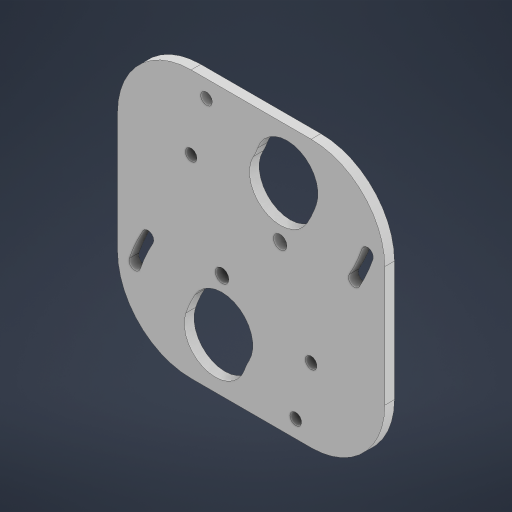
# Autodesk Inventor part: mount-plate
Saved by Autodesk Inventor 2024 (Build 280153000, 153)
## iProperties
Created: 2024-10-25
Part Number: mount-plate
Material: Generic
Document SubType Name: Modeling
Designer: loren
Density: 1 g/cm^3
Appearance: Default
Author: loren
## iProperties of the stored document mount-plate_3DPrint.ipt
Created: 2026-02-06
Part Number: mount-plate_3DPrint
Material: Generic
Document SubType Name: Modeling
Designer: lokies
Density: 1 g/cm^3
Appearance: Default
Author: lokies
Autodesk Inventor part; units mm, degrees
ref_plane "YZ Plane" through (0, 0, 0) normal (1, 0, 0) x (0, 1, 0)
ref_plane "XZ Plane" through (0, 0, 0) normal (0, 1, 0) x (-1, 0, 0)
ref_plane "XY Plane" through (0, 0, 0) normal (0, 0, 1) x (1, 0, 0)
sketch "Sketch1" plane through (0, 0, 0) normal (0, 1, 0) x (-1, 0, 0)
  line L0 (34.5, 34.5) -> (-34.5, 34.5)
  line L1 (-34.5, 34.5) -> (-34.5, -34.5)
  line L2 (-34.5, -34.5) -> (34.5, -34.5)
  line L3 (34.5, -34.5) -> (34.5, 34.5)
  point P0 (0, 0)
  point P1 (-34.5, 0)
  point P2 (0, 34.5)
  dimension "d0" = 69
  constraints: 8 end point, 2 midpoint, 2 parallel, 2 perpendicular, 1 horizontal, 1 horizontal alignment, 1 vertical alignment
  measures "d0" distance of L2.end L1.end
extrude "Extrusion1" add sketch "Sketch1" against normal blind 2.5
sketch "Sketch2" plane through (0, -2.5, 0) normal (0, -1, 0) x (1, 0, 0)
  circle A0 centre (-15.5, 15.5) radius 19.9 construction
  line L0 (-15.5, 15.5) -> (15.5, -15.5) construction
  circle A1 centre (-15.5, 15.5) radius 1.5
  circle A2 centre (-11.5216, 30.0556) radius 1.5
  line L1 (-11.5216, 30.0556) -> (28.9823, 13.2551) construction
  arc A3 (26.633, 8.4441) -> (30.0556, 16.1214) centre (-11.5216, 30.0556) ccw construction
  arc A4 (27.9381, 7.7048) -> (31.4779, 15.6448) centre (-11.5216, 30.0556) ccw
  arc A5 (25.3278, 9.1834) -> (28.6334, 16.5981) centre (-11.5216, 30.0556) ccw
  arc A6 (31.4779, 15.6448) -> (28.6334, 16.5981) centre (30.0556, 16.1214) ccw
  arc A7 (25.3278, 9.1834) -> (27.9381, 7.7048) centre (26.633, 8.4441) ccw
  arc A8 (7.5557, 19.2499) -> (9.267, 23.0885) centre (-11.5216, 30.0556) ccw construction
  arc A9 (16.8524, 20.5464) -> (1.6817, 25.6307) centre (9.267, 23.0885) ccw
  arc A10 (0.5948, 23.1927) -> (14.5166, 15.3071) centre (7.5557, 19.2499) ccw
  arc A11 (14.5166, 15.3071) -> (16.8524, 20.5464) centre (-11.5216, 30.0556) ccw
  arc A12 (0.5948, 23.1927) -> (1.6817, 25.6307) centre (-11.5216, 30.0556) ccw
  circle A13 centre (7.5557, 19.2499) radius 18.25 construction
  line L2 (-11.5216, 31.5556) -> (-11.5216, 34.5) construction
  line L3 (34.5, 34.5) -> (-34.5, 34.5) projected
  line L4 (31.5556, 16.1214) -> (34.5, 16.1214) construction
  line L5 (34.5, -34.5) -> (34.5, 34.5) projected
  line L6 (0, 0) -> (7.5, 7.5) construction
  circle A14 centre (7.5, 7.5) radius 1.75
  line L7 (7.5178, 11.25) -> (7.5083, 9.25) construction
  line L8 (-34.5, 34.5) -> (-34.5, -34.5) projected
  arc A15 (-15.5, 34.5) -> (-34.5, 15.5) centre (-15.5, 15.5) ccw
  arc A16 (34.5, 15.5) -> (15.5, 34.5) centre (15.5, 15.5) ccw
  point P0 (8.7304, 21.6553)
  dimension "d5" = 3
  dimension "d18" = 3.5
  dimension "d3" = 39.8
  dimension "d4" = 3
  dimension "d6" = 43.85
  dimension "d7" = 7
  dimension "d8" = 4
  dimension "d10" = 7
  dimension "d11" = 4
  dimension "d12" = 16
  dimension "d13" = 36.5
  dimension "d14" = 25
  dimension "d15" = 15.5
  dimension "d16" = 15.5
  dimension "d17" = 7.5
  dimension "d19" = 2
  constraints: 29 point on circle, 15 centre point, 15 coincident, 12 end point, 10 tangent, 6 point on line, 2 line through centre, 2 midpoint, 2 perpendicular, 2 vertical, 1 equal radius, 1 horizontal, 1 vertical alignment, 7 other
  measures "d3" diameter of A0
  measures "d4" diameter of A1
  measures "d6" distance of L1.start L1.end
  measures "d12" diameter of A9
  measures "d13" diameter of A13
  measures "d14" distance of point (8.73, 21.655) L0.start
  measures "d15" horizontal distance of L0.start point (0, 0)
  measures "d16" horizontal distance of point (0, 0) A1.centre
  measures "d17" horizontal distance of point (0, 0) L6.end
  measures "d19" distance of L7.start L7.end
extrude "Extrusion2" cut sketch "Sketch2" against normal through all
pattern_circular "Circular Pattern1" count 2 over 360 about axis through (0, -10, 0) along (0, 1, 0) of "Extrusion2"
equation "\"d10\" = d7"
equation "\"d11\" = d8"
equation "\"d16\" = d15"
body "Solid1"
